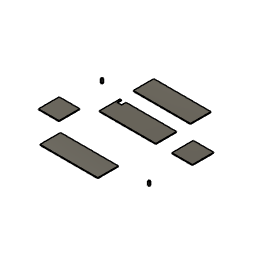
fcucover_SOURCEFILE v1 (Autodesk Fusion 360 design; units mm, degrees)
Autodesk Fusion 360 part; units mm, degrees
note: some values were not read from the file. Chosen so that the rebuilt part matches the saved one: which bodies a step acts on; which face or edge a step refers to.
sketch "Sketch1" plane through (0, 0, 0) normal (0, 0, 1) x (1, 0, 0)
  line L0 (0, 0) -> (262, 0)
  line L1 (262, 0) -> (262, 100)
  line L2 (262, 100) -> (0, 100)
  line L3 (0, 100) -> (0, 0)
  dimension "d1" = 262
  dimension "d2" = 100
  constraint horizontal L0
  constraint vertical L1
  constraint horizontal L2
  constraint vertical L3
  constraint coincident L0.start L3.end
  measures "d1" distance of L0.start L0.end
  measures "d2" distance of L0.start L2.end
extrude "Extrude1" add sketch "Sketch1" along normal blind 93 makes body 1
sketch "Sketch2" plane through (0, 0, 93) normal (0, 0, 1) x (-1, 0, 0)
  line L0 (0, -100) -> (0, 0)
  line L1 (0, 0) -> (-262, 0)
  line L2 (-262, 0) -> (-262, -100)
  line L3 (-262, -100) -> (0, -100)
  line L4 (-10, -97) -> (-259, -97)
  line L5 (-259, -97) -> (-259, -10)
  line L6 (-252, -3) -> (-3, -3)
  line L7 (-3, -3) -> (-3, -90)
  line L8 (-10, -97) -> (-10, -90)
  line L9 (-10, -90) -> (-3, -90)
  line L10 (-252, -3) -> (-252, -10)
  line L11 (-252, -10) -> (-259, -10)
  constraint horizontal L4
  constraint vertical L5
  constraint horizontal L6
  constraint vertical L7
  constraint vertical L8
  constraint horizontal L9
  constraint vertical L10
  constraint horizontal L11
extrude "Extrude2" cut sketch "Sketch2" against normal blind 90 contours L4 L5 L6 L7 L8 L9 L10 L11 bodies 1
sketch "Sketch5" plane through (0, 0, 0) normal (0, 0, -1) x (1, 0, 0)
  line L0 (0, 0) -> (0, -100)
  line L1 (0, -100) -> (262, -100)
  line L2 (262, -100) -> (262, 0)
  line L3 (262, 0) -> (0, 0)
  line L4 (10, -97) -> (30, -97)
  line L5 (30, -97) -> (30, -77)
  line L6 (30, -77) -> (10, -77)
  line L7 (10, -77) -> (10, -97)
  dimension "d14" = 20
  dimension "d15" = 20
  constraint horizontal L4
  constraint vertical L5
  constraint horizontal L6
  constraint vertical L7
  measures "d14" distance of L4.start L4.end
  measures "d15" distance of L4.start L6.end
extrude "Extrude3" cut sketch "Sketch5" against normal blind 11 contours L4 L5 L6 L7 bodies 1
split "Split1" by plane through (252, 3, 93) normal (0, 1, 0) bodies 1 makes body 2 at (184.6667, 60, 0)
move_body "Move1" bodies 1 to x (1, 0, 0) y (0, 1, 0) z (0, 0, 1) at (0, -170, 0)
split "Split2" by plane through (259, 97, 93) normal (-1, 0, 0) bodies 2 makes body 3 at (182.6667, 60, 0)
move_body "Move2" bodies 2 to x (1, 0, 0) y (0, 1, 0) z (0, 0, 1) at (70, 0, 0)
split "Split3" by plane through (10, 97, 93) normal (0, -1, 0) bodies 3 makes body 4 at (182.6667, 59, 0)
move_body "Move3" bodies 3 to x (1, 0, 0) y (0, 1, 0) z (0, 0, 1) at (0, 60, 0)
split "Split4" by plane through (3, 3, 93) normal (1, 0, 0) bodies 4 makes body 5 at (182.6667, 59, 0)
move_body "Move4" bodies 4 to x (1, 0, 0) y (0, 1, 0) z (0, 0, 1) at (-50, 0, 0)
split "Split5" by plane through (0, 0, 3) normal (0, 0, 1) bodies 5 makes body 6 at (259, 7.6667, 33) makes body 7 at (5.3333, 97, 33)
move_body "Move5" bodies 4 to x (1, 0, 0) y (0, 1, 0) z (0, 0, 1) at (0, -130, 0)
sketch "Sketch7" plane through (3, 0, 0) normal (-1, 0, 0) x (0, -1, 0)
  line L0 (-97, 3) -> (-90, 3)
  line L1 (-90, 3) -> (-90, 93)
  line L2 (-90, 93) -> (-97, 93)
  line L3 (-97, 93) -> (-97, 3)
  line L4 (-97, 3) -> (-90, 3)
  line L5 (-90, 3) -> (-90, 75)
  line L6 (-90, 75) -> (-97, 75)
  line L7 (-97, 75) -> (-97, 3)
  constraint horizontal L4
  constraint vertical L5
  constraint horizontal L6
  constraint vertical L7
  constraint coincident L1 L5.end
  constraint coincident L0.start L3.end
extrude "Extrude4" cut sketch "Sketch7" against normal blind 15 contours L0 L1 L3 L4 L5 L6 L7 bodies 7
sketch "Sketch8" plane through (252, 0, 0) normal (-1, 0, 0) x (0, -1, 0)
  line L0 (-3, 93) -> (-10, 93)
  line L1 (-10, 93) -> (-10, 3)
  line L2 (-10, 3) -> (-3, 3)
  line L3 (-3, 3) -> (-3, 93)
  line L4 (-10, 75) -> (-3, 75)
  line L5 (-3, 75) -> (-3, 3)
  line L6 (-3, 3) -> (-10, 3)
  line L7 (-10, 3) -> (-10, 75)
  constraint horizontal L4
  constraint vertical L5
  constraint horizontal L6
  constraint vertical L7
  constraint coincident L2.end L3.start
  constraint coincident L1 L4.start
extrude "Extrude5" cut sketch "Sketch8" against normal blind 20 contours L1 L2 L3 L4 L5 L6 L7 bodies 6
move_body "Move6" bodies 1 to x (1, 0, 0) y (0, 0, 1) z (0, -1, 0) at (0, -170, 170)
move_body "Move7" bodies 4 to x (0, 0, 1) y (0, 1, 0) z (-1, 0, 0) at (-50, 0, 50)
move_body "Move8" bodies 3 to x (1, 0, 0) y (0, 0, -1) z (0, 1, 0) at (0, 160, 160)
move_body "Move9" bodies 2 to x (0, 0, -1) y (0, 1, 0) z (1, 0, 0) at (332, 0, 332)
move_body "Move10" bodies 7 to x (1, 0, 0) y (0, 1, 0) z (0, 0, 1) at (0, 7, -75)
move_body "Move11" bodies 7 to x (1, 0, 0) y (0, 1, 0) z (0, 0, 1) at (-110, 21, 0)
move_body "Move12" bodies 6 to x (1, 0, 0) y (0, 1, 0) z (0, 0, 1) at (0, 0, -75)
move_body "Move13" bodies 6 to x (1, 0, 0) y (0, 1, 0) z (0, 0, 1) at (150, -180, 0)
sketch "Sketch9" plane through (0, 0, 18) normal (0, 0, 1) x (-1, 0, 0)
  line L0 (-409, 177) -> (-409, 170)
  line L1 (-409, 170) -> (-402, 170)
  line L2 (-402, 170) -> (-402, 177)
  line L3 (-402, 177) -> (-409, 177)
  circle A0 centre (103.5, -121.5) radius 0.85
  dimension "d28" = 1.7
  measures "d28" diameter of A0
extrude "Extrude6" cut sketch "Sketch9" against normal blind 16 contours A0 bodies 7
sketch "Sketch10" plane through (0, 0, 18) normal (0, 0, 1) x (-1, 0, 0)
  line L0 (-409, 177) -> (-409, 170)
  line L1 (-409, 170) -> (-402, 170)
  line L2 (-402, 170) -> (-402, 177)
  line L3 (-402, 177) -> (-409, 177)
  circle A0 centre (-405.5, 173.5) radius 0.85
  dimension "d31" = 1.7
  measures "d31" diameter of A0
extrude "Extrude7" cut sketch "Sketch10" against normal blind 16 contours A0 bodies 6
